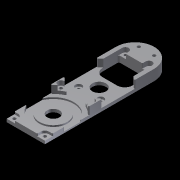
# Autodesk Inventor part: JointC3'cover_2nd
Saved by Autodesk Inventor 2011 SP1 (Build 150282100, 282)
## iProperties
Created: 2013-02-07
Part Number: JointC3'cover_2nd
Document SubType Name: Modeling
Designer: JohnHenry
Density: 1 g/cm^3
Author: JohnHenry
Autodesk Inventor part; units mm, degrees
ref_plane "YZ Plane" through (0, 0, 0) normal (1, 0, 0) x (0, 1, 0)
ref_plane "XZ Plane" through (0, 0, 0) normal (0, 1, 0) x (-1, 0, 0)
ref_plane "XY Plane" through (0, 0, 0) normal (0, 0, 1) x (1, 0, 0)
sketch "スケッチ1" plane through (0, 0, 0) normal (0, 0, 1) x (1, 0, 0)
  line L0 (-12.5, 42) -> (12.5, 42)
  line L1 (12.5, 42) -> (12.5, -42)
  line L2 (12.5, -42) -> (-12.5, -42)
  line L3 (-12.5, -42) -> (-12.5, 42)
  point P0 (0, 0)
  dimension "d0" = 25
  dimension "d1" = 84
  dimension "d2" = 42
  dimension "d3" = 12.5
  constraints: 8 end point, 2 parallel, 1 horizontal, 1 perpendicular
  measures "d0" distance between parallel lines of L3 L1
  measures "d1" distance of L2.end L0.start
  measures "d2" distance from line of L2 point (0, 0)
  measures "d3" distance from line of L1 point (0, 0)
extrude "押し出し1" add sketch "スケッチ1" along normal blind 2
sketch "スケッチ2" plane through (0, 0, 2) normal (0, 0, 1) x (1, 0, 0)
  line L0 (-12.5, 42) -> (12.5, 42) projected
  line L1 (12.5, -42) -> (-12.5, -42) projected
  line L2 (0, 42) -> (0, -42)
  point P0 (0, 0)
  point P1 (-7.7, 30.9)
  point P2 (-7.2, -0.2)
  point P3 (7.7, 30.9)
  point P4 (7.2, -0.2)
  dimension "d6" = 41.8
  dimension "d7" = 72.9
  dimension "d8" = 14.4
  dimension "d9" = 15.4
  constraints: 2 end point, 2 midpoint, 2 symmetric about line
  measures "d6" distance from line of L1 point (-7.2, -0.2)
  measures "d7" distance from line of L1 point (-7.7, 30.9)
  measures "d8" diameter of point (-7.2, -0.2) L2
  measures "d9" diameter of point (-7.7, 30.9) L2
hole "Hole1" at (-7.7, 30.9, 2) at (-7.2, -0.2, 2) at (7.2, -0.2, 2) at (7.7, 30.9, 2) direction (0, 0, -1) diameter 1.8 depth 8 tip angle 118
sketch "スケッチ3" plane through (0, 0, 2) normal (0, 0, 1) x (1, 0, 0)
  line L0 (12.5, 42) -> (12.5, -42) projected
  line L1 (12.5, -42) -> (-12.5, -42) projected
  point P0 (0, 0)
  point P1 (0, 6)
  dimension "d17" = 48
  dimension "d18" = 12.5
  measures "d17" distance from line of L1 point (0, 6)
  measures "d18" distance from line of L0 point (0, 6)
hole "Hole2" at (0, 6, 2) direction (0, 0, -1) diameter 9 depth 8 tip angle 118
sketch "スケッチ4" plane through (0, 0, 2) normal (0, 0, 1) x (1, 0, 0)
  line L0 (-12.5, 42) -> (12.5, 42) projected
  line L1 (12.5, -42) -> (-12.5, -42) projected
  line L2 (-9.85, 28.72) -> (-5.1081, 28.72)
  line L3 (9.85, 28.72) -> (9.85, 12.9)
  line L4 (9.85, 12.9) -> (-9.85, 12.9)
  line L5 (-9.85, 12.9) -> (-9.85, 28.72)
  line L6 (0, 42) -> (0, -42)
  line L7 (-5.1081, 28.72) -> (5.1081, 28.72)
  line L8 (5.1081, 28.72) -> (9.85, 28.72)
  point P0 (0, 0)
  dimension "d27" = 19.7
  dimension "d28" = 19.7
  dimension "d29" = 15.82
  dimension "d64" = 13.28
  constraints: 14 end point, 4 parallel, 3 horizontal, 3 perpendicular, 2 midpoint, 1 point on line
  measures "d27" distance between parallel lines of L5 L3
  measures "d28" diameter of L3 L6
  measures "d29" distance between parallel lines of L4 L2
  measures "d64" distance between parallel lines of L8 L0
sketch "スケッチ5" plane through (0, 0, 2) normal (0, 0, 1) x (1, 0, 0)
  line L0 (12.5, 42) -> (12.5, -42) projected
  line L1 (-12.5, -42) -> (-12.5, 42) projected
  line L2 (12.5, -42) -> (-12.5, -42) projected
  point P0 (0, 0)
  point P1 (-10, -39.5)
  point P2 (-10, -9)
  point P3 (10, -9)
  point P4 (10, -39.5)
  point P5 (5, 37)
  point P6 (-5, 37)
  dimension "d35" = 2.5
  dimension "d36" = 2.5
  dimension "d37" = 33
  dimension "d38" = 33
  dimension "d39" = 2.5
  dimension "d40" = 2.5
  dimension "d41" = 2.5
  dimension "d42" = 2.5
  dimension "d43" = 79
  dimension "d44" = 79
  dimension "d111" = 7.5
  dimension "d112" = 7.5
  measures "d35" distance from line of L2 point (10, -39.5)
  measures "d36" distance from line of L2 point (-10, -39.5)
  measures "d37" distance from line of L2 point (-10, -9)
  measures "d38" distance from line of L2 point (10, -9)
  measures "d39" distance from line of point (10, -39.5) L0
  measures "d40" distance from line of L0 point (10, -9)
  measures "d41" distance from line of L1 point (-10, -39.5)
  measures "d42" distance from line of L1 point (-10, -9)
  measures "d43" distance from line of L2 point (5, 37)
  measures "d44" distance from line of L2 point (-5, 37)
  measures "d111" distance from line of L0 point (5, 37)
  measures "d112" distance from line of L1 point (-5, 37)
hole "Hole3" at (-10, -39.5, 2) at (-10, -9, 2) at (10, -9, 2) at (10, -39.5, 2) at (5, 37, 2) at (-5, 37, 2) direction (0, 0, -1) diameter 2.1 end through all
sketch "スケッチ6" plane through (0, 0, 2) normal (0, 0, 1) x (1, 0, 0)
  line L0 (12.5, 42) -> (12.5, -42) projected
  line L1 (12.5, -42) -> (-12.5, -42) projected
  point P0 (0, 0)
  point P1 (0, -24)
  dimension "d54" = 12.5
  dimension "d55" = 18
  measures "d54" distance from line of L0 point (0, -24)
  measures "d55" distance from line of L1 point (0, -24)
hole "Hole4" at (0, -24, 2) direction (0, 0, -1) diameter 8 end through all
fillet "フィレット2" radius 12.5 2 edges at (-12.5, 42, 1) (12.5, 42, 1)
extrude "押し出し3" cut sketch "スケッチ4" against normal through all
fillet "フィレット3" radius 5.05 2 edges at (-9.85, 12.9, 1) (9.85, 12.9, 1)
fillet "フィレット4" radius 1.05 2 edges at (-9.85, 28.72, 1) (9.85, 28.72, 1)
sketch "スケッチ7" plane through (0, 0, 2) normal (0, 0, 1) x (1, 0, 0)
  line L0 (-9.85, 17.95) -> (-9.85, 27.67) projected
  arc A0 (-8.8, 28.72) -> (-9.85, 27.67) centre (-8.8, 27.67) ccw projected
  line L1 (-8.8, 28.72) -> (8.8, 28.72) projected
  arc A1 (9.85, 27.67) -> (8.8, 28.72) centre (8.8, 27.67) ccw projected
  line L2 (9.85, 27.67) -> (9.85, 17.95) projected
  arc A2 (12.5, 29.5) -> (-12.5, 29.5) centre (0, 29.5) ccw projected
  line L3 (-12.5, -42) -> (-12.5, 29.5) projected
  line L4 (12.5, -42) -> (-12.5, -42) projected
  line L5 (12.5, 29.5) -> (12.5, -42) projected
  circle A3 centre (-5, 37) radius 1.05 projected
  circle A4 centre (5, 37) radius 1.05 projected
  circle A5 centre (10, -39.5) radius 1.05 projected
  circle A6 centre (10, -9) radius 1.05 projected
  circle A7 centre (-10, -9) radius 1.05 projected
  circle A8 centre (-10, -39.5) radius 1.05 projected
  circle A9 centre (7.7, 30.9) radius 0.9 projected
  circle A10 centre (-7.7, 30.9) radius 0.9 projected
  arc A11 (5.5678, -9) -> (12.5, -3.9875) centre (0, 6) ccw
  arc A12 (-5.5678, -9) -> (-12.5, -14.0125) centre (0, -24) ccw
  arc A13 (5.5678, -9) -> (-5.5678, -9) centre (0, -24) ccw
  arc A14 (-5.5678, -9) -> (5.5678, -9) centre (0, 6) ccw
  arc A15 (9.85, 18.6086) -> (-9.85, 18.6086) centre (0, 6) ccw
  arc A16 (-9.85, 18.6086) -> (-12.5, 15.9875) centre (0, 6) ccw
  arc A17 (-12.5, 15.9875) -> (-12.5, -3.9875) centre (0, 6) ccw
  arc A18 (12.5, 15.9875) -> (9.85, 18.6086) centre (0, 6) ccw
  arc A19 (12.5, -3.9875) -> (12.5, 15.9875) centre (0, 6) ccw
  arc A20 (-12.5, -3.9875) -> (-5.5678, -9) centre (0, 6) ccw
  arc A21 (-12.5, -14.0125) -> (-12.5, -33.9875) centre (0, -24) ccw
  arc A22 (-12.5, -33.9875) -> (12.5, -33.9875) centre (0, -24) ccw
  arc A23 (12.5, -14.0125) -> (5.5678, -9) centre (0, -24) ccw
  arc A24 (12.5, -33.9875) -> (12.5, -14.0125) centre (0, -24) ccw
  point P0 (0, 0)
  dimension "d69" = 32
  dimension "d70" = 32
  constraints: 28 point on circle, 14 centre point, 10 point on line
  measures "d69" diameter of A11
  measures "d70" diameter of A12
extrude "押し出し4" add sketch "スケッチ7" along normal blind 5 contours A16 L3 A2 L5 A18 L2 A1 L1 A0 L0 | A20 A12 L3 | L5 A23 A11
fillet "フィレット5" radius 0.5 8 edges at (12.5, -14.0125, 4.5) (12.5, -3.9875, 4.5) (12.5, 15.9875, 4.5) (-12.5, 15.9875, 4.5) (-12.5, -3.9875, 4.5) (-12.5, -14.0125, 4.5) (-5.5678, -9, 4.5) (5.5678, -9, 4.5)
sketch "スケッチ8" plane through (0, 0, 7) normal (0, 0, 1) x (1, 0, 0)
  point P0 (0, 0)
  point P1 (-7.7, 30.9)
  point P2 (7.7, 30.9)
hole "Hole5" at (-7.7, 30.9, 7) at (7.7, 30.9, 7) direction (0, 0, -1) diameter 4.3 depth 3
sketch "スケッチ10" plane through (0, 0, 7) normal (0, 0, 1) x (1, 0, 0)
  line L0 (-12.5, -12.6752) -> (-12.5, -5.3248) projected
  point P0 (0, 0)
  point P1 (-10, -9)
  dimension "d113" = 9
  dimension "d114" = 2.5
  measures "d113" vertical distance of point (0, 0) point (-10, -9)
  measures "d114" distance from line of L0 point (-10, -9)
hole "Hole7" at (-10, -9, 7) direction (0, 0, -1) diameter 4.2 depth 3
sketch "スケッチ11" plane through (0, 0, 7) normal (0, 0, 1) x (1, 0, 0)
  line L0 (12.5, -5.3248) -> (12.5, -12.6752) projected
  point P0 (0, 0)
  point P1 (10, -9)
  dimension "d115" = 9
  dimension "d117" = 2.5
  measures "d115" vertical distance of point (10, -9) point (0, 0)
  measures "d117" distance from line of point (10, -9) L0
hole "Hole8" at (10, -9, 7) direction (0, 0, -1) diameter 4.2 depth 3
sketch "スケッチ14" plane through (0, 0, 7) normal (0, 0, 1) x (1, 0, 0)
  circle A0 centre (7.7, 30.9) radius 2.15 projected
  circle A1 centre (-7.7, 30.9) radius 2.15 projected
  circle A2 centre (-7.7, 30.9) radius 2.15 projected
  line L0 (-9.85, 30.9) -> (-5.55, 30.9)
  line L1 (-5.55, 30.9) -> (-5.55, 27.667)
  line L2 (-5.55, 27.667) -> (-9.85, 27.667)
  line L3 (-9.85, 27.667) -> (-9.85, 30.9)
  line L4 (5.55, 30.9) -> (9.85, 30.9)
  line L5 (9.85, 30.9) -> (9.85, 27.67)
  line L6 (9.85, 27.67) -> (5.55, 27.67)
  line L7 (5.55, 27.67) -> (5.55, 30.9)
  point P0 (0, 0)
  dimension "d135" = 0
  dimension "d136" = 2.15
  dimension "d137" = 4.3
  constraints: 16 end point, 4 parallel, 3 horizontal alignment, 2 horizontal, 2 perpendicular, 3 other
  measures "d135" distance from line of L0 point (-7.7, 30.9)
  measures "d136" distance of point (-7.7, 30.9) L0.end
  measures "d137" distance of L4.start L4.end
extrude "押し出し7" cut sketch "スケッチ14" against normal blind 3 contours L5 L6 L7 A0 | A0 L4 | L1 L2 L3 A1 | A1 L0 picked at (7.7864, 30.1886) picked at (-7.6136, 30.1886)
sketch "スケッチ15" plane through (0, 0, 7) normal (0, 0, 1) x (1, 0, 0)
  arc A0 (-8.4426, -10.4087) -> (-8.4426, -7.5913) centre (-10, -9) ccw projected
  arc A1 (-6.6656, -9.4545) -> (-8.4426, -10.4087) centre (0, -24) ccw projected
  arc A2 (-6.6656, -9.4545) -> (-6.6656, -8.5455) centre (-6.8739, -9) ccw projected
  arc A3 (-8.4426, -7.5913) -> (-6.6656, -8.5455) centre (0, 6) ccw projected
  point P0 (0, 0)
extrude "押し出し8" cut sketch "スケッチ15" against normal blind 3
sketch "スケッチ16" plane through (0, 0, 7) normal (0, 0, 1) x (1, 0, 0)
  arc A0 (8.4426, -7.5913) -> (8.4426, -10.4087) centre (10, -9) ccw projected
  arc A1 (6.6656, -8.5455) -> (8.4426, -7.5913) centre (0, 6) ccw projected
  arc A2 (6.6656, -8.5455) -> (6.6656, -9.4545) centre (6.8739, -9) ccw projected
  arc A3 (8.4426, -10.4087) -> (6.6656, -9.4545) centre (0, -24) ccw projected
  point P0 (0, 0)
extrude "押し出し9" cut sketch "スケッチ16" against normal blind 3
fillet "フィレット9" radius 0.2 4 edges at (9.2986, -7.0206, 5.5) (9.2986, -10.9794, 5.5) (-9.2986, -10.9794, 5.5) (-9.2986, -7.0206, 5.5)
sketch "スケッチ17" plane through (0, 0, 2) normal (0, 0, 1) x (1, 0, 0)
  circle A0 centre (0, -24) radius 9.15
  circle A1 centre (0, -24) radius 13.35
  point P0 (0, 0)
  dimension "d127" = 18.3
  dimension "d128" = 26.7
  constraints: 2 centre point
  measures "d127" diameter of A0
  measures "d128" diameter of A1
extrude "押し出し10" cut sketch "スケッチ17" against normal blind 1
fillet "フィレット10" radius 0.2 4 edges at (-12.5, -28.6875, 1.5) (-12.5, -19.3125, 1.5) (12.5, -19.3125, 1.5) (12.5, -28.6875, 1.5)
sketch "スケッチ18" plane through (0, 0, 2) normal (0, 0, 1) x (1, 0, 0)
  arc A0 (12.5, -29.6844) -> (12.1185, -29.6005) centre (12.3, -29.6844) ccw projected
  arc A1 (-12.1185, -29.6005) -> (12.1185, -29.6005) centre (0, -24) ccw projected
  arc A2 (-12.1185, -29.6005) -> (-12.5, -29.6844) centre (-12.3, -29.6844) ccw projected
  line L0 (-12.5, -29.6844) -> (-12.5, -42) projected
  line L1 (12.5, -29.6844) -> (12.5, -42) projected
  circle A3 centre (-10, -39.5) radius 2.5
  line L2 (12.5, -42) -> (-12.5, -42) projected
  circle A4 centre (10, -39.5) radius 2.5
  line L3 (10, -37) -> (12.5, -37)
  line L4 (7.5, -39.5) -> (7.5, -42)
  line L5 (-7.5, -39.5) -> (-7.5, -42)
  line L6 (-10, -37) -> (-12.5, -37)
  point P0 (0, 0)
  constraints: 8 end point, 6 tangent, 4 perpendicular, 4 point on circle, 4 point on line, 2 centre point
extrude "押し出し11" add sketch "スケッチ18" along normal blind 1.5 contours L1 L3 A4 L4 L2 L5 A3 L6 L0 A2 A1 A0
fillet "フィレット11" radius 0.5 4 edges at (-12.5, -37, 2.75) (-7.5, -42, 2.75) (7.5, -42, 2.75) (12.5, -37, 2.75)
fillet "フィレット12" radius 0.5 2 edges at (-5.55, 28.72, 5.5) (5.55, 28.72, 5.5)
sketch "スケッチ19" plane through (0, 0, 2) normal (0, 0, 1) x (1, 0, 0)
  circle A0 centre (-7.2, -0.2) radius 0.9 projected
  circle A1 centre (7.2, -0.2) radius 0.9 projected
  point P0 (0, 0)
  constraints: 2 coincident
hole "Hole9" at (-7.2, -0.2, 2) at (7.2, -0.2, 2) direction (0, 0, -1) diameter 4.2 depth 1.5
equation "\"d2\" = 0.5 * d1"
equation "\"d3\" = 0.5 * d0"
equation "\"d28\" = d27"
equation "\"d36\" = d35"
equation "\"d37\" = d38"
equation "\"d39\" = d35"
equation "\"d40\" = d35"
equation "\"d41\" = d35"
equation "\"d42\" = d35"
equation "\"d44\" = d43"
equation "\"d112\" = d111"
equation "\"d137\" = 2 * d136"
